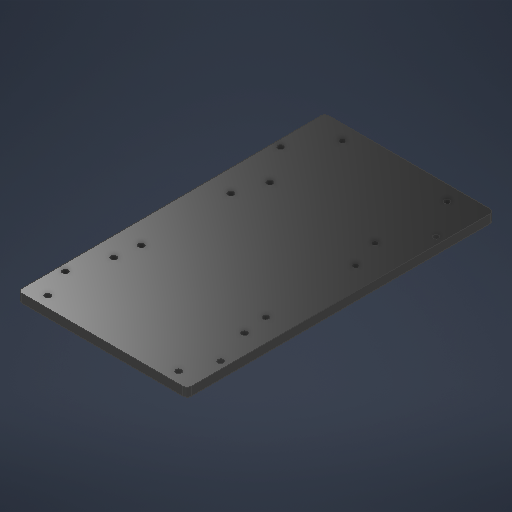
# Autodesk Inventor part: BASE_ELETRONICA
Saved by Autodesk Inventor 2027.1 (Build 311270010, 270A)
## iProperties
Created: 2026-08-16
Part Number: BASE_ELETRONICA
Material: Genérico
Document SubType Name: Modeling
Designer: Evellyn
Density: 1 g/cm^3
Appearance: Padrão
Author: Evellyn
Autodesk Inventor part; units mm, degrees
ref_plane "YZ Plane" through (0, 0, 0) normal (1, 0, 0) x (0, 1, 0)
ref_plane "XZ Plane" through (0, 0, 0) normal (0, 1, 0) x (-1, 0, 0)
ref_plane "XY Plane" through (0, 0, 0) normal (0, 0, 1) x (1, 0, 0)
sketch "Esboço1" plane through (0, 0, 0) normal (0, 1, 0) x (-1, 0, 0)
  line L0 (-38, -70) -> (38, -70)
  line L1 (40, -68) -> (40, 73)
  line L2 (38, 75) -> (-38, 75)
  line L3 (-40, 73) -> (-40, -68)
  line L4 (-40, -70) -> (40, 75) construction
  line L5 (40, -70) -> (-40, 75) construction
  line L6 (0, 77.1224) -> (0, -77.4589)
  line L7 (55.8999, -0.1682) -> (-68.6929, -0.1682)
  arc A0 (40, 73) -> (38, 75) centre (38, 73) ccw
  arc A1 (-38, 75) -> (-40, 73) centre (-38, 73) ccw
  arc A2 (-40, -68) -> (-38, -70) centre (-38, -68) ccw
  arc A3 (38, -70) -> (40, -68) centre (38, -68) ccw
  line L8 (-33, 36.5618) -> (33, 36.5618)
  line L9 (33, 36.5618) -> (33, 71.9618)
  line L10 (33, 71.9618) -> (-33, 71.9618)
  line L11 (-33, 71.9618) -> (-33, 36.5618)
  line L12 (-33, 36.5618) -> (33, 71.9618) construction
  line L13 (33, 36.5618) -> (-33, 71.9618) construction
  line L14 (-35.75, -19.4382) -> (35.75, -19.4382)
  line L15 (35.75, -19.4382) -> (35.75, 31.5618)
  line L16 (35.75, 31.5618) -> (-35.75, 31.5618)
  line L17 (-35.75, 31.5618) -> (-35.75, -19.4382)
  line L18 (-35.75, -19.4382) -> (35.75, 31.5618) construction
  line L19 (35.75, -19.4382) -> (-35.75, 31.5618) construction
  line L20 (-27.1, -67.2382) -> (27.1, -67.2382)
  line L21 (29.1, -65.2382) -> (29.1, -26.4382)
  line L22 (27.1, -24.4382) -> (-27.1, -24.4382)
  line L23 (-29.1, -26.4382) -> (-29.1, -65.2382)
  line L24 (-29.1, -67.2382) -> (29.1, -24.4382) construction
  line L25 (29.1, -67.2382) -> (-29.1, -24.4382) construction
  arc A4 (29.1, -26.4382) -> (27.1, -24.4382) centre (27.1, -26.4382) ccw
  arc A5 (27.1, -67.2382) -> (29.1, -65.2382) centre (27.1, -65.2382) ccw
  arc A6 (-29.1, -65.2382) -> (-27.1, -67.2382) centre (-27.1, -65.2382) ccw
  arc A7 (-27.1, -24.4382) -> (-29.1, -26.4382) centre (-27.1, -26.4382) ccw
  circle A8 centre (30.85, 69.8118) radius 1.35
  circle A9 centre (-30.85, 69.8118) radius 1.35
  circle A10 centre (30.85, 38.7118) radius 1.35
  circle A11 centre (-30.85, 38.7118) radius 1.35
  circle A12 centre (29.4, 27.2118) radius 1.35
  circle A13 centre (-29.4, 27.2118) radius 1.35
  circle A14 centre (29.4, -15.0882) radius 1.35
  circle A15 centre (-29.4, -15.0882) radius 1.35
  line L26 (29.1, -45.8382) -> (-29.1, -45.8382)
  circle A16 centre (24.75, -28.7882) radius 1.35
  circle A17 centre (-24.75, -28.7882) radius 1.35
  circle A18 centre (24.75, -62.8882) radius 1.35
  circle A19 centre (-24.75, -62.8882) radius 1.35
  circle A20 centre (36.65, 55.7814) radius 1.35
  circle A21 centre (-36.65, 55.7814) radius 1.35
  circle A22 centre (36.65, -45.8382) radius 1.35
  circle A23 centre (-36.65, -45.8382) radius 1.35
  point P0 (0, 54.2618)
  point P1 (0, 6.0618)
  point P2 (0, -45.8382)
  dimension "d0" = 80
  dimension "d1" = 145
  dimension "d8" = 2
  dimension "d12" = 66
  dimension "d13" = 35.4
  dimension "d14" = 71.5
  dimension "d15" = 51
  dimension "d16" = 58.2
  dimension "d17" = 42.8
  dimension "d18" = 5
  dimension "d19" = 5
  dimension "d20" = 2
  dimension "d21" = 2.7
  dimension "d22" = 0.8
  dimension "d23" = 0.8
  dimension "d24" = 2.7
  dimension "d25" = 3
  dimension "d26" = 5
  dimension "d27" = 2.7
  dimension "d28" = 3
  dimension "d30" = 3
  dimension "d33" = 2.7
  dimension "d34" = 2
  dimension "d35" = 2.7
  dimension "d36" = 2
  dimension "d44" = 22.1618
  dimension "d45" = 3.35
  dimension "d46" = 17.2186
  constraints: 54 end point, 24 centre point, 19 point on line, 16 point on circle, 16 tangent, 8 midpoint, 8 parallel, 7 symmetric about line, 6 equal radius, 5 horizontal, 4 perpendicular, 1 vertical, 7 other
  measures "d0" distance of L5.end L4.end
  measures "d1" distance of L4.end L5.start
  measures "d8" radius of A0
  measures "d12" distance of L10.end L9.end
  measures "d13" distance of L9.end L8.end
  measures "d14" distance of L16.end L15.end
  measures "d15" distance of L15.end L14.end
  measures "d16" distance of L25.end L24.end
  measures "d17" distance of L24.end L25.start
  measures "d18" distance between parallel lines of L16 L8
  measures "d19" distance between parallel lines of L14 L22
  measures "d20" radius of A4
  measures "d21" diameter of A8
  measures "d22" distance edge to line of A8 L9
  measures "d23" distance edge to line of A8 L10
  measures "d24" diameter of A12
  measures "d25" distance edge to line of A12 L16
  measures "d26" distance edge to line of A12 L15
  measures "d27" diameter of A16
  measures "d28" distance edge to line of A16 L21
  measures "d30" distance edge to line of A16 L22
  measures "d33" diameter of A20
  measures "d34" distance edge to line of A20 L1
  measures "d35" diameter of A22
  measures "d36" distance edge to line of A22 L1
  measures "d44" vertical distance of A23.centre A2.centre
  measures "d45" distance from line of A23.centre L3
  measures "d46" vertical distance of A1.centre A21.centre
extrude "Extrusão1" add sketch "Esboço1" along normal blind 4 contours A2 L3 L7 L17 L14 L6 L22 A7 L23 A6 L20 L0 | L6 L20 A5 L21 A4 L22 L14 L15 L7 L1 A3 L0 | L20 A6 L23 L26 L6 | L6 L26 L21 A5 L20 | L3 A1 L2 L6 L10 L11 L8 L16 L17 L7 | L26 L23 A7 L22 L6 | L6 L22 A4 L21 L26 | L17 L16 L6 L7 | L7 L6 L14 L17 | L7 L15 L16 L6 L8 L9 L10 L2 A0 L1 | L7 L15 L14 L6 | L6 L16 L15 L7 | L10 L9 L8 L6 | L6 L8 L11 L10 | A20 | A21 | A22 | A23
hole "Furo1" at (36.65, 0, -45.8382) at (-36.65, 0, -45.8382) at (-36.65, 0, 55.7814) at (36.65, 0, 55.7814) direction (0, 1, 0) diameter 2.7 end through all
